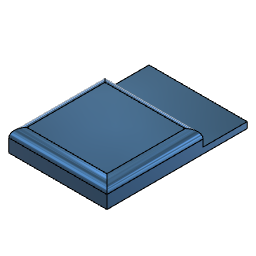
BMD-300 v3 (Autodesk Fusion 360 design; units mm, degrees)
Autodesk Fusion 360 part; units mm, degrees
sketch "Sketch1" plane through (0, 0, 0) normal (0, 1, 0) x (1, 0, 0)
  line L0 (0, 0) -> (9.8, 0)
  line L1 (9.8, 0) -> (9.8, 14)
  line L2 (9.8, 14) -> (0, 14)
  line L3 (0, 14) -> (0, 0)
  line L4 (0, 9.6) -> (9.8, 9.6)
  dimension "d1" = 9.8
  dimension "d2" = 14
  dimension "d3" = 9.6
  constraint horizontal L0
  constraint vertical L1
  constraint horizontal L2
  constraint vertical L3
  constraint coincident L0.start L3.end
  constraint coincident L3 L4.start
  constraint coincident L1 L4.end
  constraint perpendicular L1 L4
  measures "d1" distance of L0.start L0.end
  measures "d2" distance of L0.start L2.end
  measures "d3" distance of L0 L4
extrude "Extrude1" add sketch "Sketch1" along normal blind 0.6
extrude "Extrude2" add sketch "Sketch1" along normal blind 2.2 contours L0 L1 L3 L4
fillet "Fillet1" radius 0.9 4 edges at (4.9, 2.2, -9.6) (0, 2.2, -4.8) (4.9, 2.2, 0) (9.8, 2.2, -4.8)
named bodies: "BMD-300"
